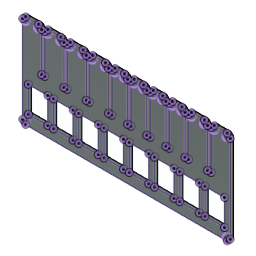
kerf comb (Autodesk Fusion 360 design; units mm, degrees)
Autodesk Fusion 360 part; units mm, degrees
sketch "Sketch1" plane through (0, 0, 0) normal (0, 1, 0) x (1, 0, 0)
  line L0 (-97, 45) -> (97, 45)
  line L1 (100, 42) -> (100, -42)
  line L2 (97, -45) -> (-97, -45)
  line L3 (-100, -42) -> (-100, 42)
  line L4 (-100, 45) -> (100, -45) construction
  line L5 (100, 45) -> (-100, -45) construction
  arc A0 (-100, -42) -> (-97, -45) centre (-97, -42) ccw
  arc A1 (97, -45) -> (100, -42) centre (97, -42) ccw
  arc A2 (100, 42) -> (97, 45) centre (97, 42) ccw
  arc A3 (-97, 45) -> (-100, 42) centre (-97, 42) ccw
  line L6 (-94.4444, 10) -> (-75.6944, 10)
  line L7 (-75.6944, 10) -> (-75.6944, 35)
  line L8 (-75.6944, 35) -> (-94.4444, 35)
  line L9 (-94.4444, 35) -> (-94.4444, 10)
  line L10 (-70.1389, 10) -> (-51.3889, 10)
  line L11 (-70.1389, 35) -> (-70.1389, 10)
  line L12 (-51.3889, 10) -> (-51.3889, 35)
  line L13 (-51.3889, 35) -> (-70.1389, 35)
  line L14 (-45.8333, 10) -> (-27.0833, 10)
  line L15 (-45.8333, 35) -> (-45.8333, 10)
  line L16 (-27.0833, 10) -> (-27.0833, 35)
  line L17 (-27.0833, 35) -> (-45.8333, 35)
  line L18 (-21.5278, 10) -> (-2.7778, 10)
  line L19 (-21.5278, 35) -> (-21.5278, 10)
  line L20 (-2.7778, 10) -> (-2.7778, 35)
  line L21 (-2.7778, 35) -> (-21.5278, 35)
  line L22 (2.7778, 10) -> (21.5278, 10)
  line L23 (2.7778, 35) -> (2.7778, 10)
  line L24 (21.5278, 10) -> (21.5278, 35)
  line L25 (21.5278, 35) -> (2.7778, 35)
  line L26 (27.0833, 10) -> (45.8333, 10)
  line L27 (27.0833, 35) -> (27.0833, 10)
  line L28 (45.8333, 10) -> (45.8333, 35)
  line L29 (45.8333, 35) -> (27.0833, 35)
  line L30 (51.3889, 10) -> (70.1389, 10)
  line L31 (51.3889, 35) -> (51.3889, 10)
  line L32 (70.1389, 10) -> (70.1389, 35)
  line L33 (70.1389, 35) -> (51.3889, 35)
  line L34 (75.6944, 10) -> (94.4444, 10)
  line L35 (75.6944, 35) -> (75.6944, 10)
  line L36 (94.4444, 10) -> (94.4444, 35)
  line L37 (94.4444, 35) -> (75.6944, 35)
  line L38 (-81.58, -45) -> (-78.58, -45)
  line L39 (-78.58, -45) -> (-78.58, -4.5)
  line L40 (-78.58, -4.5) -> (-81.58, -4.5)
  line L41 (-81.58, -4.5) -> (-81.58, -45)
  line L42 (-60.16, -45) -> (-57.11, -45)
  line L43 (-57.11, -45) -> (-57.11, -4.5)
  line L44 (-57.11, -4.5) -> (-60.16, -4.5)
  line L45 (-60.16, -4.5) -> (-60.16, -45)
  line L46 (-38.69, -45) -> (-35.59, -45)
  line L47 (-35.59, -45) -> (-35.59, -4.5)
  line L48 (-35.59, -4.5) -> (-38.69, -4.5)
  line L49 (-38.69, -4.5) -> (-38.69, -45)
  line L50 (-17.17, -45) -> (-14.02, -45)
  line L51 (-14.02, -45) -> (-14.02, -4.5)
  line L52 (-14.02, -4.5) -> (-17.17, -4.5)
  line L53 (-17.17, -4.5) -> (-17.17, -45)
  line L54 (4.4, -45) -> (1.2, -45)
  line L55 (1.2, -45) -> (1.2, -4.5)
  line L56 (1.2, -4.5) -> (4.4, -4.5)
  line L57 (4.4, -4.5) -> (4.4, -45)
  line L58 (19.62, -45) -> (22.87, -45)
  line L59 (22.87, -45) -> (22.87, -4.5)
  line L60 (22.87, -4.5) -> (19.62, -4.5)
  line L61 (19.62, -4.5) -> (19.62, -45)
  line L62 (56.41, -45) -> (59.76, -45)
  line L63 (59.76, -45) -> (59.76, -4.5)
  line L64 (59.76, -4.5) -> (56.41, -4.5)
  line L65 (56.41, -4.5) -> (56.41, -45)
  line L66 (78.18, -45) -> (81.58, -45)
  line L67 (81.58, -45) -> (81.58, -4.5)
  line L68 (81.58, -4.5) -> (78.18, -4.5)
  line L69 (78.18, -4.5) -> (78.18, -45)
  line L70 (37.99, -45) -> (41.29, -45)
  line L71 (41.29, -45) -> (41.29, -4.5)
  line L72 (41.29, -4.5) -> (37.99, -4.5)
  line L73 (37.99, -4.5) -> (37.99, -45)
  line L74 (-100, -24.75) -> (-81.58, -24.75) construction
  line L75 (-57.11, -24.75) -> (-38.69, -24.75) construction
  line L76 (-35.59, -24.75) -> (-17.17, -24.75) construction
  line L77 (-14.02, -24.75) -> (4.4, -24.75) construction
  line L78 (1.2, -24.75) -> (19.62, -24.75) construction
  line L79 (22.87, -24.75) -> (41.29, -24.75) construction
  line L80 (37.99, -24.75) -> (56.41, -24.75) construction
  line L81 (59.76, -24.75) -> (78.18, -24.75) construction
  line L82 (81.58, -24.75) -> (100, -24.75) construction
  line L83 (-78.58, -24.75) -> (-60.16, -24.75) construction
  dimension "d8" = 3
  dimension "d9" = 90
  dimension "d10" = 200
  dimension "d16" = 5.5556
  dimension "d17" = 10
  dimension "d18" = 10
  dimension "d19" = 18.75
  dimension "d22" = 24.3056
  dimension "d23" = 0
  dimension "d24" = 3
  dimension "d25" = 40.5
  dimension "d26" = 3.05
  dimension "d27" = 3.1
  dimension "d28" = 3.15
  dimension "d29" = 3.2
  dimension "d30" = 3.25
  dimension "d31" = 3.3
  dimension "d32" = 3.35
  dimension "d33" = 3.4
  constraint horizontal L0
  constraint perpendicular L0 L1
  constraint parallel L0 L2
  constraint parallel L1 L3
  constraint coincident L4 origin
  constraint coincident L5 origin
  constraint coincident L5.end L2
  constraint coincident L5.end L3
  constraint tangent L2 A0
  constraint tangent L3 A0
  constraint coincident L4.end L2
  constraint coincident L4.end L1
  constraint tangent L2 A1
  constraint tangent L1 A1
  constraint equal A0 A1
  constraint coincident L5.start L1
  constraint coincident L5.start L0
  constraint tangent L1 A2
  constraint tangent L0 A2
  constraint equal A0 A2
  constraint coincident L4.start L0
  constraint coincident L4.start L3
  constraint tangent L0 A3
  constraint tangent L3 A3
  constraint equal A0 A3
  constraint horizontal L6
  constraint vertical L7
  constraint horizontal L8
  constraint vertical L9
  constraint horizontal L38
  constraint vertical L39
  constraint horizontal L40
  constraint vertical L41
  constraint coincident L2 L38.start
  constraint horizontal L42
  constraint vertical L43
  constraint horizontal L44
  constraint vertical L45
  constraint coincident L2 L42.start
  constraint horizontal L46
  constraint vertical L47
  constraint horizontal L48
  constraint vertical L49
  constraint coincident L2 L46.start
  constraint horizontal L50
  constraint vertical L51
  constraint horizontal L52
  constraint vertical L53
  constraint coincident L2 L50.start
  constraint horizontal L54
  constraint vertical L55
  constraint horizontal L56
  constraint vertical L57
  constraint coincident L2 L54.start
  constraint horizontal L58
  constraint vertical L59
  constraint horizontal L60
  constraint vertical L61
  constraint coincident L2 L58.start
  constraint horizontal L62
  constraint vertical L63
  constraint horizontal L64
  constraint vertical L65
  constraint coincident L2 L62.start
  constraint horizontal L66
  constraint vertical L67
  constraint horizontal L68
  constraint vertical L69
  constraint coincident L2 L66.start
  constraint horizontal L70
  constraint vertical L71
  constraint horizontal L72
  constraint vertical L73
  constraint coincident L2 L70.start
  constraint collinear L40 L44
  constraint collinear L44 L48
  constraint collinear L48 L52
  constraint collinear L52 L56
  constraint collinear L56 L60
  constraint collinear L60 L72
  constraint collinear L64 L72
  constraint collinear L64 L68
  constraint coincident L3 L74.start
  constraint midpoint L41 L74.end
  constraint coincident L43 L75.start
  constraint coincident L49 L75.end
  constraint coincident L47 L76.start
  constraint coincident L53 L76.end
  constraint coincident L51 L77.start
  constraint coincident L57 L77.end
  constraint coincident L55 L78.start
  constraint coincident L61 L78.end
  constraint coincident L59 L79.start
  constraint coincident L71 L79.end
  constraint coincident L73 L80.start
  constraint coincident L65 L80.end
  constraint coincident L63 L81.start
  constraint coincident L69 L81.end
  constraint parallel L79 L81
  constraint coincident L67 L82.start
  constraint coincident L1 L82.end
  constraint perpendicular L1 L82
  constraint coincident L39 L83.start
  constraint coincident L45 L83.end
  constraint perpendicular L45 L83
  constraint collinear L74 L83
  constraint collinear L75 L83
  constraint collinear L75 L76
  constraint collinear L76 L77
  constraint collinear L77 L78
  constraint collinear L78 L79
  constraint collinear L79 L80
  constraint collinear L80 L81
  constraint collinear L81 L82
  constraint equal L81 L82
  constraint equal L80 L81
  constraint equal L79 L80
  constraint equal L78 L79
  constraint equal L77 L78
  constraint equal L76 L77
  constraint equal L75 L76
  constraint equal L74 L75
  constraint equal L74 L83
  measures "d8" radius of A0
  measures "d9" distance of L0 L2
  measures "d10" distance of L1 L3
  measures "d16" distance of L3 L9
  measures "d17" distance of L0 L8
  measures "d18" distance of origin L6
  measures "d19" distance of L7.end L8.end
  measures "d24" distance of L39.end L40.end
  measures "d25" distance of L38.start L40.end
  measures "d26" distance of L43.end L44.end
  measures "d27" distance of L47.end L48.end
  measures "d28" distance of L51.end L52.end
  measures "d29" distance of L55.end L56.end
  measures "d30" distance of L59.end L60.end
  measures "d31" distance of L71.end L72.end
  measures "d32" distance of L63.end L64.end
  measures "d33" distance of L67.end L68.end
extrude "Extrude1" add sketch "Sketch1" along normal blind 3 contours L0 L1 L2 L3 A0 A1 A2 A3 L39 L40 L41 L43 L44 L45 L47 L48 L49 L51 L52 L53 L55 L56 L57 L59 L60 L61 L63 L64 L65 L67 L68 L69 L71 L72 L73
fillet "Fillet1" radius 3 18 edges at (-81.58, 1.5, 45) (-78.58, 1.5, 45) (-60.16, 1.5, 45) (-57.11, 1.5, 45) (-35.59, 1.5, 45) (-38.69, 1.5, 45) (-14.02, 1.5, 45) (-17.17, 1.5, 45) (1.2, 1.5, 45) (4.4, 1.5, 45) (19.62, 1.5, 45) (22.87, 1.5, 45) (37.99, 1.5, 45) (41.29, 1.5, 45) (56.41, 1.5, 45) (59.76, 1.5, 45) (78.18, 1.5, 45) (81.58, 1.5, 45)
sketch "Sketch2" plane through (0, 0, 0) normal (0, -1, 0) x (1, 0, 0)
  line L0 (94.4444, -35) -> (75.6944, -35)
  line L1 (75.6944, -35) -> (75.6944, -10)
  line L2 (75.6944, -10) -> (94.4444, -10)
  line L3 (94.4444, -10) -> (94.4444, -35)
  line L4 (-94.4444, -35) -> (-94.4444, -10)
  line L5 (-94.4444, -10) -> (-75.6944, -10)
  line L6 (-75.6944, -10) -> (-75.6944, -35)
  line L7 (-75.6944, -35) -> (-94.4444, -35)
  line L8 (70.1389, -35) -> (51.3889, -35)
  line L9 (51.3889, -35) -> (51.3889, -10)
  line L10 (51.3889, -10) -> (70.1389, -10)
  line L11 (70.1389, -10) -> (70.1389, -35)
  line L12 (-2.7778, -35) -> (-21.5278, -35)
  line L13 (-21.5278, -35) -> (-21.5278, -10)
  line L14 (-21.5278, -10) -> (-2.7778, -10)
  line L15 (-2.7778, -10) -> (-2.7778, -35)
  line L16 (21.5278, -35) -> (2.7778, -35)
  line L17 (2.7778, -35) -> (2.7778, -10)
  line L18 (2.7778, -10) -> (21.5278, -10)
  line L19 (21.5278, -10) -> (21.5278, -35)
  line L20 (-51.3889, -35) -> (-70.1389, -35)
  line L21 (-70.1389, -35) -> (-70.1389, -10)
  line L22 (-70.1389, -10) -> (-51.3889, -10)
  line L23 (-51.3889, -10) -> (-51.3889, -35)
  line L24 (-27.0833, -35) -> (-45.8333, -35)
  line L25 (-45.8333, -35) -> (-45.8333, -10)
  line L26 (-45.8333, -10) -> (-27.0833, -10)
  line L27 (-27.0833, -10) -> (-27.0833, -35)
  line L28 (45.8333, -35) -> (27.0833, -35)
  line L29 (27.0833, -35) -> (27.0833, -10)
  line L30 (27.0833, -10) -> (45.8333, -10)
  line L31 (45.8333, -10) -> (45.8333, -35)
  arc A0 (84.58, 45) -> (81.58, 42) centre (84.58, 42) ccw
  line L32 (81.58, 42) -> (81.58, 4.5)
  line L33 (81.58, 4.5) -> (78.18, 4.5)
  line L34 (78.18, 4.5) -> (78.18, 42)
  arc A1 (78.18, 42) -> (75.18, 45) centre (75.18, 42) ccw
  line L35 (75.18, 45) -> (62.76, 45)
  arc A2 (62.76, 45) -> (59.76, 42) centre (62.76, 42) ccw
  line L36 (59.76, 42) -> (59.76, 4.5)
  line L37 (59.76, 4.5) -> (56.41, 4.5)
  line L38 (56.41, 4.5) -> (56.41, 42)
  arc A3 (56.41, 42) -> (53.41, 45) centre (53.41, 42) ccw
  line L39 (53.41, 45) -> (44.29, 45)
  arc A4 (44.29, 45) -> (41.29, 42) centre (44.29, 42) ccw
  line L40 (41.29, 42) -> (41.29, 4.5)
  line L41 (41.29, 4.5) -> (37.99, 4.5)
  line L42 (37.99, 4.5) -> (37.99, 42)
  arc A5 (37.99, 42) -> (34.99, 45) centre (34.99, 42) ccw
  line L43 (34.99, 45) -> (25.87, 45)
  arc A6 (25.87, 45) -> (22.87, 42) centre (25.87, 42) ccw
  line L44 (22.87, 42) -> (22.87, 4.5)
  line L45 (22.87, 4.5) -> (19.62, 4.5)
  line L46 (19.62, 4.5) -> (19.62, 42)
  arc A7 (19.62, 42) -> (16.62, 45) centre (16.62, 42) ccw
  line L47 (16.62, 45) -> (7.4, 45)
  arc A8 (7.4, 45) -> (4.4, 42) centre (7.4, 42) ccw
  line L48 (4.4, 42) -> (4.4, 4.5)
  line L49 (4.4, 4.5) -> (1.2, 4.5)
  line L50 (1.2, 4.5) -> (1.2, 42)
  arc A9 (1.2, 42) -> (-1.8, 45) centre (-1.8, 42) ccw
  line L51 (-1.8, 45) -> (-11.02, 45)
  arc A10 (-11.02, 45) -> (-14.02, 42) centre (-11.02, 42) ccw
  line L52 (-14.02, 42) -> (-14.02, 4.5)
  line L53 (-14.02, 4.5) -> (-17.17, 4.5)
  line L54 (-17.17, 4.5) -> (-17.17, 42)
  arc A11 (-17.17, 42) -> (-20.17, 45) centre (-20.17, 42) ccw
  line L55 (-20.17, 45) -> (-32.59, 45)
  arc A12 (-32.59, 45) -> (-35.59, 42) centre (-32.59, 42) ccw
  line L56 (-35.59, 42) -> (-35.59, 4.5)
  line L57 (-35.59, 4.5) -> (-38.69, 4.5)
  line L58 (-38.69, 4.5) -> (-38.69, 42)
  arc A13 (-38.69, 42) -> (-41.69, 45) centre (-41.69, 42) ccw
  line L59 (-41.69, 45) -> (-54.11, 45)
  arc A14 (-54.11, 45) -> (-57.11, 42) centre (-54.11, 42) ccw
  line L60 (-57.11, 42) -> (-57.11, 4.5)
  line L61 (-57.11, 4.5) -> (-60.16, 4.5)
  line L62 (-60.16, 4.5) -> (-60.16, 42)
  arc A15 (-60.16, 42) -> (-63.16, 45) centre (-63.16, 42) ccw
  line L63 (-63.16, 45) -> (-75.58, 45)
  arc A16 (-75.58, 45) -> (-78.58, 42) centre (-75.58, 42) ccw
  line L64 (-78.58, 42) -> (-78.58, 4.5)
  line L65 (-78.58, 4.5) -> (-81.58, 4.5)
  line L66 (-81.58, 4.5) -> (-81.58, 42)
  arc A17 (-81.58, 42) -> (-84.58, 45) centre (-84.58, 42) ccw
  line L67 (-84.58, 45) -> (-97, 45)
  arc A18 (-97, 45) -> (-100, 42) centre (-97, 42) ccw
  line L68 (-100, 42) -> (-100, -42)
  arc A19 (-100, -42) -> (-97, -45) centre (-97, -42) ccw
  line L69 (-97, -45) -> (97, -45)
  arc A20 (97, -45) -> (100, -42) centre (97, -42) ccw
  line L70 (100, -42) -> (100, 42)
  arc A21 (100, 42) -> (97, 45) centre (97, 42) ccw
  line L71 (97, 45) -> (84.58, 45)
equation "Wbox = 200 mm" comment "Width of bounding box"
equation "Hbox = 90 mm" comment "Height of box"
equation "Thickness = 3 mm" comment "Thickness of stock used"
equation "Kerfincrement = 0.05 mm" comment "the value with which the kerf is increased"
equation "Diameter = 5 mm" comment "Dia of hole"
equation "Fillet = 3 mm" comment "Fillet around bouding box"
equation "Kerfsteps = 6 mm"
equation "d8 = Fillet"
equation "d9 = Hbox"
equation "d10 = Wbox"
equation "PScount = 8" comment "No of power boxes"
equation "PSwidth = ( Wbox * 0.75 ) / PScount" comment "powerbox width"
equation "PSgap = ( Wbox - ( PSwidth * PScount ) ) / ( PScount + 1 )" comment "gap b/w power boxes"
equation "d16 = PSgap"
equation "d17 = Wbox * 0.05"
equation "d18 = Wbox * 0.05"
equation "d19 = PSwidth"
equation "d20 = PScount"
equation "d22 = PSwidth + PSgap"
equation "d24 = Thickness"
equation "d25 = 0.45 * Hbox"
equation "d26 = Thickness + ( 1 * Kerfincrement )"
equation "d27 = Thickness + ( 2 * Kerfincrement )"
equation "d28 = Thickness + ( 3 * Kerfincrement )"
equation "d29 = Thickness + ( 4 * Kerfincrement )"
equation "d30 = Thickness + ( 5 * Kerfincrement )"
equation "d31 = Thickness + ( 6 * Kerfincrement )"
equation "d32 = Thickness + ( 7 * Kerfincrement )"
equation "d33 = Thickness + ( 8 * Kerfincrement )"
equation "d34 = Thickness"
equation "d37 = Fillet"
